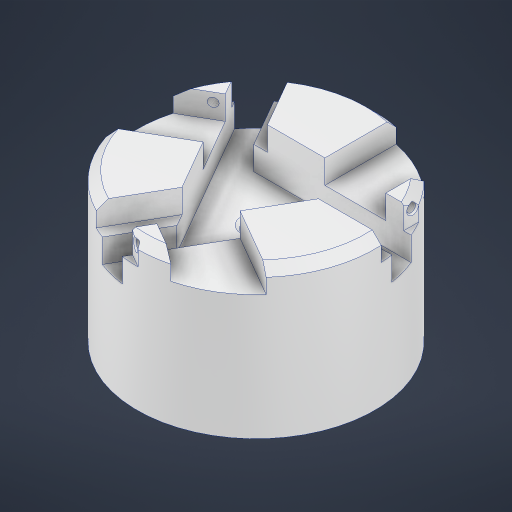
# Autodesk Inventor part: BaseSupport
Saved by Autodesk Inventor 2023 (Build 270158000, 158)
## iProperties
Created: 2023-02-24
Part Number: BaseSupport
Material: Aluminum 6061
Document SubType Name: Modeling
Designer: roota
Density: 2.7 g/cm^3
Appearance: Aluminum - Flat
Mass: 612.501 g
Surface Area: 232.858 cm^2
Volume: 226.852 cm^3
Author: roota
Autodesk Inventor part; units mm, degrees
ref_plane "YZ Plane" through (0, 0, 0) normal (1, 0, 0) x (0, 1, 0)
ref_plane "XZ Plane" through (0, 0, 0) normal (0, 1, 0) x (-1, 0, 0)
ref_plane "XY Plane" through (0, 0, 0) normal (0, 0, 1) x (1, 0, 0)
sketch "Sketch1" plane through (0, 0, 0) normal (0, 1, 0) x (-1, 0, 0)
  circle A0 centre (0, 0) radius 70 construction
  line L0 (32.262182, 28.381545) -> (0.406888, 28.381545) construction
  line L1 (0.406888, 28.381545) -> (0.406888, 1.427614) construction
  line L2 (0.406888, 1.427614) -> (32.262182, 1.427614) construction
  line L3 (32.262182, 1.427614) -> (32.262182, 28.381545) construction
  line L4 (21.414213, 1.427614) -> (78.161879, 1.427614) construction
  line L5 (78.161879, 1.427614) -> (78.161879, -1.51684) construction
  line L6 (78.161879, -1.51684) -> (21.414213, -1.51684) construction
  line L7 (21.414213, -1.51684) -> (21.414213, 1.427614) construction
  line L8 (8.448048, -42.130641) -> (24.375695, -14.543148) construction
  line L9 (24.375695, -14.543148) -> (1.032906, -1.066182) construction
  line L10 (1.032906, -1.066182) -> (-14.894741, -28.653676) construction
  line L11 (-14.894741, -28.653676) -> (8.448048, -42.130641) construction
  line L12 (-9.470757, -19.25906) -> (-37.844589, -68.40398) construction
  line L13 (-37.844589, -68.40398) -> (-40.394561, -66.931753) construction
  line L14 (-40.394561, -66.931753) -> (-12.020728, -17.786833) construction
  line L15 (-12.020728, -17.786833) -> (-9.470757, -19.25906) construction
  line L16 (-40.71023, 13.749097) -> (-24.782583, -13.838397) construction
  line L17 (-24.782583, -13.838397) -> (-1.439794, -0.361432) construction
  line L18 (-1.439794, -0.361432) -> (-17.367441, 27.226062) construction
  line L19 (-17.367441, 27.226062) -> (-40.71023, 13.749097) construction
  line L20 (-11.943457, 17.831446) -> (-40.31729, 66.976366) construction
  line L21 (-40.31729, 66.976366) -> (-37.767318, 68.448593) construction
  line L22 (-37.767318, 68.448593) -> (-9.393485, 19.303673) construction
  line L23 (-9.393485, 19.303673) -> (-11.943457, 17.831446) construction
  circle A1 centre (0, 0) radius 40
  dimension "d0" = 140
  dimension "d3" = 360
  dimension "d5" = 80
  constraints: 48 end point, 6 coincident, 4 parallel, 3 point on line, 2 centre point, 2 horizontal, 2 perpendicular, 53 other
  measures "d0" diameter of A0
  measures "d5" diameter of A1
extrude "Extrusion1" add sketch "Sketch1" along normal blind 50
sketch "Sketch4" plane through (0, 50, 0) normal (0, 1, 0) x (1, 0, 0)
  line L0 (8, 2.2) -> (52.769682, 2.2)
  line L1 (52.769682, 2.2) -> (52.769682, 51.677795)
  line L2 (52.769682, 51.677795) -> (8, 51.677795)
  line L3 (8, 51.677795) -> (8, 2.2)
  point P0 (0, 0)
  point P1 (-40, 0)
  point P2 (-40, 0)
  dimension "d25" = 8
  dimension "d26" = 32.8
  constraints: 8 end point, 2 parallel, 1 horizontal, 1 perpendicular
  measures "d25" distance from line of point (0, 0) L3
extrude "Extrusion3" cut sketch "Sketch4" against normal blind 8
sketch "Sketch5" plane through (0, 50, 0) normal (0, 1, 0) x (1, 0, 0)
  circle A0 centre (0, 0) radius 15.2
  dimension "d30" = 30.4
  constraints: 1 centre point, 1 coincident
  measures "d30" diameter of A0
extrude "Extrusion4" cut sketch "Sketch5" against normal blind 16
sketch "Sketch6" plane through (0, 42, 0) normal (0, 1, 0) x (1, 0, 0)
  line L0 (0, 6.2) -> (49.649635, 6.2)
  line L1 (49.649635, 6.2) -> (49.649635, 15.2)
  line L2 (49.649635, 15.2) -> (0, 15.2)
  line L3 (0, 15.2) -> (0, 6.2)
  line L4 (39.939454, 2.2) -> (15.039947, 2.2)
  line L5 (8, 12.924396) -> (8, 39.191836)
  line L6 (0, 0) -> (15.2, 0)
  line L7 (15.2, 0) -> (15.2, 6.2)
  line L8 (15.2, 6.2) -> (0, 6.2)
  line L9 (0, 6.2) -> (0, 0)
  point P0 (0, 0)
  point P1 (8, 35)
  dimension "d33" = 9
  dimension "d34" = 4
  dimension "d39" = 15.2
  constraints: 16 end point, 4 parallel, 2 horizontal, 2 perpendicular, 1 coincident, 1 point on line, 1 vertical alignment
  measures "d33" distance of L0.end L1.end
  measures "d34" distance between parallel lines of L4 L0
  measures "d39" distance from line of point (0, 0) L7
extrude "Extrusion5" cut sketch "Sketch6" along normal blind 20.75 and the other way blind 8
pattern_circular "Circular Pattern2" count 3 over 360 about axis through (0, 0, 0) along (0, 1, 0) of "Extrusion3", "Extrusion5"
sketch "Sketch7" plane through (0, 50, 0) normal (0, 1, 0) x (1, 0, 0)
  line L0 (8, 15.2) -> (36.999459, 15.2)
  arc A0 (39.939454, 2.2) -> (39.516579, 6.2) centre (0, 0) ccw
  line L1 (8, 15.2) -> (8, 39.191836)
  arc A1 (-31.663316, 24.442472) -> (-37.941125, -12.667715) centre (0, 0) ccw
  line L2 (-17.163586, -0.671797) -> (-37.941125, -12.667715)
  line L3 (-31.663316, 24.442472) -> (-17.163586, -0.671797)
  arc A2 (-5.336144, -39.642472) -> (29.941125, -26.524121) centre (0, 0) ccw
  line L4 (9.163586, -14.528203) -> (29.941125, -26.524121)
  line L5 (-5.336144, -39.642472) -> (9.163586, -14.528203)
  line L6 (28.5, 28.066884) -> (28.5, 15.2)
  line L7 (0, 15.2) -> (36.999459, 15.2)
  line L8 (34.5, 15.2) -> (34.5, 20.242282)
  arc A3 (36.999459, 15.2) -> (8, 39.191836) centre (0, 0) ccw
  line L9 (15.2, 6.2) -> (15.2, 2.2)
  line L10 (39.939454, 2.2) -> (15.2, 2.2)
  line L11 (39.516579, 6.2) -> (15.2, 6.2)
  arc A4 (-18.064471, -35.688582) -> (-14.388932, -37.322361) centre (0, 0) ccw
  line L12 (-2.230642, -16.263586) -> (-14.388932, -37.322361)
  line L13 (-5.694744, -14.263586) -> (-2.230642, -16.263586)
  line L14 (-18.064471, -35.688582) -> (-5.694744, -14.263586)
  point P0 (28.5, 28.066884)
  dimension "d43" = 20.5
  dimension "d46" = 6
  constraints: 4 end point, 2 perpendicular, 2 point on circle, 2 point on line
  measures "d43" distance between parallel lines of L1 L6
  measures "d46" distance between parallel lines of L6 L8
extrude "Extrusion6" add sketch "Sketch7" along normal blind 8 from surface at -8 contours L6 A3 L8 L0 | L10 L9 L11 A0
sketch "Sketch8" plane through (34.5, 50, -15.2) normal (1, 0, 0) x (0, 0, -1)
  circle A0 centre (3, -3) radius 1.5
  line L0 (0, 0) -> (5.042282, 0)
  line L1 (0, -8) -> (0, 0)
  point P0 (-15.2, -50)
  dimension "d47" = 3
  dimension "d51" = 3
  dimension "d84" = 3
  constraints: 1 centre point
  measures "d47" diameter of A0
  measures "d51" distance from line of L0 A0.centre
  measures "d84" distance from line of A0.centre L1
extrude "Extrusion7" cut sketch "Sketch8" against normal blind 10
thread "Thread1" size "M3x0.5" class "6H" standard "ISO Metric profile" length 15
extrude "Extrusion8" cut sketch "Sketch7" against normal up to surface (16 mm away) contours L8 A3 L0 | L10 L9 L11 A0
pattern_circular "Circular Pattern3" count 3 over 360 about axis through (0, 0, 0) along (0, 1, 0)
sketch "Sketch9" plane through (0, 50, 0) normal (0, 1, 0) x (1, 0, 0)
  line L0 (26.327172, 15.2) -> (-26.327172, 15.2)
  line L1 (-26.327172, 15.2) -> (0, -30.4)
  line L2 (0, -30.4) -> (26.327172, 15.2)
  line L3 (-1.086414, -32.281724) -> (9.163586, -14.528203)
  line L4 (-27.413586, 17.081724) -> (-17.163586, -0.671797)
  point P0 (0, 0)
  point P1 (0, 15.2)
  point P2 (-13.163586, -7.6)
  point P3 (13.163586, -7.6)
  constraints: 6 end point, 3 midpoint, 2 point on line, 1 horizontal
extrude "Extrusion9" cut sketch "Sketch9" against normal up to surface (16 mm away)
sketch "Sketch10" plane through (0, 34, 0) normal (0, 1, 0) x (1, 0, 0)
  circle A0 centre (0, 0) radius 4
  dimension "d61" = 8
  constraints: 1 centre point, 1 coincident
  measures "d61" diameter of A0
extrude "Extrusion10" cut sketch "Sketch10" against normal blind 41.25
thread "Thread2" size "M8x1.25" class "6H" standard "ANSI Metric M Profile" length 15
chamfer "Chamfer2" distance 1 angle 45 1 edges at (-4, 34, 0)
chamfer "Chamfer3" distance 0.5 angle 45 3 edges at (34.5, 47, -16.7) (-2.7874, 47, 38.2279) (-31.7126, 47, -21.5279)
chamfer "Chamfer4" distance 3 angle 45 6 edges at (37.7769, 50, 13.1494) (5.2082, 50, 39.6595) (-30.2762, 50, 26.141) (-36.9502, 50, -15.3193) (-7.5007, 50, -39.2904) (31.742, 50, -24.3402)
sketch "Sketch12" plane through (0, 0, 0) normal (0, -1, 0) x (1, 0, 0)
  circle A0 centre (0, 0) radius 25 construction
  point P0 (-25, 0)
  point P1 (0, 25)
  point P2 (25, 0)
  point P3 (0, -25)
  dimension "d76" = 50
  constraints: 4 point on circle, 2 horizontal alignment, 2 vertical alignment, 1 centre point, 1 coincident
  measures "d76" diameter of A0
hole "Hole2" at (-25, 0, 0) at (0, 0, -25) at (25, 0, 0) at (0, 0, 25) direction (0, 1, 0) diameter 4.134 depth 14.2 tip angle 118 thread size "M5x0.8" class "6H" standard "ISO Metric profile"
body "Solid1"
